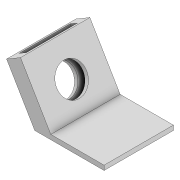
# Autodesk Inventor part: vtail_wing_piece
Saved by Autodesk Inventor 2022 (Build 260153000, 153)
## iProperties
Created: 2022-05-19
Part Number: vtail_wing_piece
Material: Generic
Document SubType Name: Modeling
Designer: Thomas
Density: 1 g/cm^3
Appearance: Default
Author: Thomas
Autodesk Inventor part; units mm, degrees
ref_plane "YZ Plane" through (0, 0, 0) normal (1, 0, 0) x (0, 1, 0)
ref_plane "XZ Plane" through (0, 0, 0) normal (0, 1, 0) x (-1, 0, 0)
ref_plane "XY Plane" through (0, 0, 0) normal (0, 0, 1) x (1, 0, 0)
sketch "Sketch1" plane through (0, 0, 0) normal (0, 0, 1) x (1, 0, 0)
  line L0 (0, 0) -> (30, 0)
  line L1 (0, 0) -> (-12.1809, 20.6791)
  line L2 (0, 0) -> (24, 0) construction
  line L3 (-12.1809, 20.6791) -> (-6.1495, 24.2319)
  line L4 (30, 0) -> (30, 2)
  line L5 (30, 2) -> (6.9461, 2)
  line L6 (6.9461, 2) -> (-6.1495, 24.2319)
  dimension "d0" = 30
  dimension "d1" = 24
  dimension "d2" = 120.5
  dimension "d3" = 7
  dimension "d4" = 2
  constraints: 14 end point, 3 perpendicular, 2 horizontal, 1 equal length, 1 vertical
  measures "d0" distance of L0.start L0.end
  measures "d1" distance of L0.start L1.end
  measures "d2" angle of L2 L1
  measures "d3" distance of L1.end L3.end
  measures "d4" distance of L0.end L4.end
extrude "Extrusion1" add sketch "Sketch1" along normal blind 30
sketch "Sketch2" plane through (-12.1809, 20.6791, 30) normal (-0.5075384, 0.8616292, 0) x (0.8616292, 0.5075384, 0)
  line L0 (1.75, 26) -> (5.25, 26)
  line L1 (5.25, 26) -> (5.25, 4)
  line L2 (5.25, 4) -> (1.75, 4)
  line L3 (1.75, 4) -> (1.75, 26)
  line L4 (7, 30) -> (7, 0) projected
  line L5 (0, 30) -> (0, 0) projected
  line L6 (7, 0) -> (0, 0) projected
  line L7 (7, 30) -> (0, 30) projected
  dimension "d7" = 22
  dimension "d8" = 3.5
  dimension "d9" = 7
  dimension "d10" = 30
  dimension "d11" = 4
  dimension "d12" = 1.75
  constraints: 8 end point, 2 parallel, 1 horizontal, 1 perpendicular
  measures "d7" distance of L0.end L1.end
  measures "d8" distance of L1.end L2.end
  measures "d9" distance between parallel lines of L4 L5
  measures "d10" distance between parallel lines of L6 L7
  measures "d11" distance between parallel lines of L0 L7
  measures "d12" distance between parallel lines of L5 L3
extrude "Extrusion2" cut sketch "Sketch2" against normal through all contours L0 L1 L2 L3
sketch "Sketch3" plane through (0, 0, 0) normal (-0.8616292, -0.5075384, 0) x (0, 0, 1)
  circle A0 centre (15, 10) radius 6.5
  line L0 (30, 24) -> (30, 0) projected
  line L1 (0, 24) -> (0, 0) projected
  line L2 (0, 24) -> (30, 24) projected
  dimension "d15" = 13
  dimension "d16" = 30
  dimension "d17" = 15
  dimension "d18" = 14
  constraints: 1 centre point
  measures "d15" diameter of A0
  measures "d16" distance between parallel lines of L0 L1
  measures "d17" distance from line of L1 A0.centre
  measures "d18" distance from line of L2 A0.centre
extrude "Extrusion3" cut sketch "Sketch3" against normal through all
equation "\"d11\" = -0.5 * d7 + 0.5 * d10"
equation "\"d12\" = -0.5 * d8 + 0.5 * d9"
equation "\"d17\" = 0.5 * d16"
body "Solid1"
